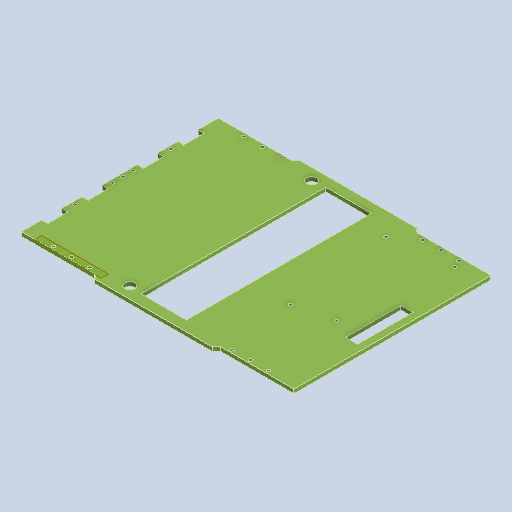
# Autodesk Inventor part: верхняя пластина
Saved by Autodesk Inventor 2024.2 (Build 282272000, 272)
## iProperties
Created: 2025-11-23
Part Number: верхняя пластина
Material: Типовые
Document SubType Name: Modeling
Designer: katya_notebook
Density: 1 g/cm^3
Appearance: Оливково-зеленый
Mass: 177.745 g
Surface Area: 959.322 cm^2
Volume: 177.745 cm^3
Author: katya_notebook
Autodesk Inventor part; units mm, degrees
ref_plane "YZ Plane" through (0, 0, 0) normal (1, 0, 0) x (0, 1, 0)
ref_plane "XZ Plane" through (0, 0, 0) normal (0, 1, 0) x (-1, 0, 0)
ref_plane "XY Plane" through (0, 0, 0) normal (0, 0, 1) x (1, 0, 0)
ref_plane "РабПлоскость1" through (-487.5503, -280.3956, -187.6025) normal (0, -1, 0) x (1, 0, 0)
sketch "Эскиз1" plane through (-487.5503, -280.3956, -187.6025) normal (0, -1, 0) x (1, 0, 0)
  line L0 (-76.4763, 6.5) -> (193.5237, 6.5)
  line L1 (193.5237, 6.5) -> (193.5237, -188.5)
  line L2 (193.5237, -188.5) -> (-76.4763, -188.5)
  line L3 (-76.4763, -188.5) -> (-76.4763, 6.5)
  line L4 (-76.4763, -188.5) -> (-76.4763, -168.5) projected
  circle A0 centre (-12, 3.25) radius 1.75
  circle A1 centre (-48, 3.25) radius 1.75
  circle A2 centre (-30, 3.25) radius 1.75
  line L5 (-76.4763, -91) -> (193.5237, -91)
  circle A3 centre (-12, -185.25) radius 1.75
  circle A4 centre (-48, -185.25) radius 1.75
  circle A5 centre (-30, -185.25) radius 1.75
  point P0 (487.5503, 187.6025)
  point P1 (-60, 3.25)
  dimension "d0" = 195
  dimension "d1" = 270
  dimension "d2" = 0
  dimension "d5" = 3.5
  dimension "d6" = 3.5
  dimension "d8" = 12
  dimension "d9" = 3.25
  dimension "d10" = 3.25
  dimension "d11" = 3.5
  dimension "d12" = 3.25
  dimension "d13" = 18
  dimension "d14" = 97.5
  constraints: 10 end point, 6 centre point, 3 symmetric about line, 2 parallel, 2 perpendicular, 1 horizontal, 1 midpoint, 1 point on line, 3 other
  measures "d0" distance of L0.end L1.end
  measures "d1" distance of L1.end L2.end
  measures "d2" distance between parallel lines of L4 L3
  measures "d5" diameter of A1
  measures "d6" diameter of A0
  measures "d8" distance of A1.centre point (-60, 3.25)
  measures "d9" distance from line of L0 A0.centre
  measures "d10" distance from line of L0 A1.centre
  measures "d11" diameter of A2
  measures "d12" distance from line of L0 A2.centre
  measures "d13" distance of A1.centre A2.centre
  measures "d14" distance between parallel lines of L5 L0
extrude "Выдавливание1" add sketch "Эскиз1" along normal blind 4 contours L0 L1 L5 L3 | L5 L1 L2 L3 | A0 | A1 | A2 | A3 | A4 | A5
sketch "Эскиз2" plane through (-487.5503, -284.3956, -187.6025) normal (0, -1, 0) x (1, 0, 0)
  circle A0 centre (-48, -185.25) radius 1.75 projected
  circle A1 centre (-30, -185.25) radius 1.75 projected
  circle A2 centre (-12, -185.25) radius 1.75 projected
  line L0 (0, -182) -> (-60, -182) projected
  line L1 (-60, -182) -> (-60, -188.5) projected
  line L2 (0, -188.5) -> (-60, -188.5) projected
  line L3 (0, -182) -> (0, -188.5) projected
  circle A3 centre (-48, 3.25) radius 1.75 projected
  circle A4 centre (-30, 3.25) radius 1.75 projected
  circle A5 centre (-12, 3.25) radius 1.75 projected
  line L4 (0, 0) -> (-60, 0) projected
  line L5 (0, 0) -> (0, 6.5) projected
  line L6 (0, 6.5) -> (-60, 6.5) projected
  line L7 (-60, 0) -> (-60, 6.5) projected
  circle A6 centre (165.0475, 3.25) radius 1.75 projected
  circle A7 centre (129.0475, 3.25) radius 1.75 projected
  circle A8 centre (147.0475, 3.25) radius 1.75 projected
  line L8 (116.803, 6.5) -> (116.803, 0) projected
  line L9 (116.803, 0) -> (176.803, 0) projected
  line L10 (176.803, 0) -> (176.803, 6.5) projected
  line L11 (176.803, 6.5) -> (116.803, 6.5) projected
  circle A9 centre (165.0475, -185.25) radius 1.75 projected
  circle A10 centre (129.0475, -185.25) radius 1.75 projected
  circle A11 centre (147.0475, -185.25) radius 1.75 projected
  line L12 (116.803, -188.5) -> (116.803, -182) projected
  line L13 (176.803, -188.5) -> (116.803, -188.5) projected
  line L14 (176.803, -182) -> (176.803, -188.5) projected
  line L15 (116.803, -182) -> (176.803, -182) projected
  line L16 (81.0237, 0.5) -> (81.0237, -182.5) projected
  line L17 (36.0237, 0.5) -> (81.0237, 0.5) projected
  line L18 (36.0237, -182.5) -> (36.0237, 0.5) projected
  line L19 (36.0237, -182.5) -> (81.0237, -182.5) projected
  point P0 (487.5503, 187.6025)
extrude "Выдавливание2" cut sketch "Эскиз2" against normal blind 10 contours A0 | A1 | A2 | A3 | A4 | A5 | A6 | A7 | A8 | A9 | A10 | A11
sketch "Эскиз3" plane through (-487.5503, -284.3956, -187.6025) normal (0, -1, 0) x (1, 0, 0)
  circle A0 centre (23.5237, -1) radius 5 projected
  circle A1 centre (23.5237, -181) radius 5 projected
  line L0 (36.0237, -182.5) -> (36.0237, 0.5) projected
  line L1 (81.0237, 0.5) -> (81.0237, -182.5) projected
  line L2 (36.0237, 0.5) -> (81.0237, 0.5) projected
  line L3 (81.0237, -182.5) -> (36.0237, -182.5) projected
  point P0 (487.5503, 187.6025)
extrude "Выдавливание3" cut sketch "Эскиз3" against normal blind 10
sketch "Эскиз4" plane through (-487.5503, -284.3956, -187.6025) normal (0, -1, 0) x (1, 0, 0)
  arc A0 (116.803, 10.7701) -> (120.803, 6.5) centre (124.2371, 13.7254) ccw projected
  line L0 (116.803, 10.7701) -> (0.2701, 10.7701) projected
  arc A1 (-4, 6.5) -> (0.2701, 10.7701) centre (-7.1034, 13.8735) ccw projected
  arc A2 (0, -192.5) -> (-4, -188.5) centre (-7.2915, -195.7915) ccw projected
  line L1 (0, -192.5) -> (116.803, -192.5) projected
  arc A3 (120.803, -188.5) -> (116.803, -192.5) centre (124.0945, -195.7915) ccw projected
  line L2 (120.803, -188.5) -> (-4, -188.5)
  line L3 (-4, 6.5) -> (120.803, 6.5)
  point P0 (487.5503, 187.6025)
  constraints: 4 end point, 1 horizontal, 1 parallel
extrude "Выдавливание4" add sketch "Эскиз4" against normal blind 4
sketch "Эскиз5" plane through (-487.5503, -284.3956, -187.6025) normal (0, -1, 0) x (1, 0, 0)
  line L0 (174.5237, -118.4235) -> (174.5237, -63.4235) projected
  line L1 (186.5237, -118.4235) -> (174.5237, -118.4235) projected
  line L2 (186.5237, -63.4235) -> (186.5237, -118.4235) projected
  line L3 (174.5237, -63.4235) -> (186.5237, -63.4235) projected
  point P0 (487.5503, 187.6025)
extrude "Выдавливание5" cut sketch "Эскиз5" against normal blind 10
sketch "Эскиз6" plane through (-487.5503, -284.3956, -187.6025) normal (0, -1, 0) x (1, 0, 0)
  circle A0 centre (155.9244, -73.304) radius 1.7 projected
  circle A1 centre (119.3724, -64.137) radius 1.7 projected
  circle A2 centre (108.4264, -169.57) radius 1.7 projected
  circle A3 centre (168.1164, -177.698) radius 1.7 projected
  point P0 (487.5503, 187.6025)
extrude "Выдавливание6" cut sketch "Эскиз6" against normal blind 10
ref_plane "РабПлоскость2" through (-558.0266, -285.3956, -376.1025) normal (1, 0, 0) x (0, 1, 0)
sketch "Эскиз7" plane through (-564.0266, -280.3956, -376.1025) normal (-1, 0, 0) x (0, 0, 1)
  line L0 (175, -5) -> (175, 0) projected
  line L1 (155, 0) -> (155, -5) projected
  line L2 (155, -5) -> (175, -5) projected
  line L3 (195, 0) -> (0, 0) projected
  line L4 (115, -5) -> (135, -5) projected
  line L5 (135, -5) -> (135, 0) projected
  line L6 (115, 0) -> (115, -5) projected
  line L7 (80, -5) -> (80, 0) projected
  line L8 (60, -5) -> (80, -5) projected
  line L9 (60, 0) -> (60, -5) projected
  line L10 (40, -5) -> (40, 0) projected
  line L11 (20, -5) -> (40, -5) projected
  line L12 (20, 0) -> (20, -5) projected
  line L13 (95.75, 39.705) -> (95.75, 46.205) projected
  line L14 (88.875, 55.705) -> (88.875, 49.205) projected
  line L15 (88.875, 49.205) -> (90.375, 49.205) projected
  line L16 (90.375, 49.205) -> (90.375, 46.205) projected
  line L17 (90.375, 46.205) -> (88.875, 46.205) projected
  line L18 (88.875, 39.705) -> (85.375, 39.705) projected
  line L19 (85.375, 39.705) -> (85.375, 46.205) projected
  line L20 (85.375, 46.205) -> (83.875, 46.205) projected
  line L21 (83.875, 46.205) -> (83.875, 49.205) projected
  line L22 (83.875, 49.205) -> (85.375, 49.205) projected
  line L23 (85.375, 49.205) -> (85.375, 55.705) projected
  line L24 (80, 59.705) -> (80, 60.705) projected
  line L25 (80, 60.705) -> (60, 60.705) projected
  line L26 (60, 60.705) -> (60, 59.705) projected
  line L27 (51.75, 55.705) -> (51.75, 49.205) projected
  line L28 (51.75, 49.205) -> (53.25, 49.205) projected
  line L29 (53.25, 49.205) -> (53.25, 46.205) projected
  line L30 (53.25, 46.205) -> (51.75, 46.205) projected
  line L31 (51.75, 39.705) -> (48.25, 39.705) projected
  line L32 (48.25, 39.705) -> (48.25, 46.205) projected
  line L33 (48.25, 46.205) -> (46.75, 46.205) projected
  line L34 (46.75, 46.205) -> (46.75, 49.205) projected
  line L35 (46.75, 49.205) -> (48.25, 49.205) projected
  line L36 (48.25, 49.205) -> (48.25, 55.705) projected
  line L37 (40, 59.705) -> (40, 60.705) projected
  line L38 (40, 60.705) -> (20, 60.705) projected
  line L39 (20, 60.705) -> (20, 59.705) projected
  line L40 (0, 55.705) -> (0, 0) projected
  line L41 (20, 0) -> (0, 0) projected
  line L42 (20, 0) -> (20, -5) projected
  line L43 (20, -5) -> (40, -5) projected
  line L44 (40, -5) -> (40, 0) projected
  line L45 (48.25, 0) -> (40, 0) projected
  line L46 (48.25, 0) -> (48.25, 6.5) projected
  line L47 (48.25, 6.5) -> (46.75, 6.5) projected
  line L48 (46.75, 6.5) -> (46.75, 9.5) projected
  line L49 (46.75, 9.5) -> (48.25, 9.5) projected
  line L50 (48.25, 9.5) -> (48.25, 16) projected
  line L51 (48.25, 16) -> (51.75, 16) projected
  line L52 (51.75, 16) -> (51.75, 9.5) projected
  line L53 (51.75, 9.5) -> (53.25, 9.5) projected
  line L54 (53.25, 9.5) -> (53.25, 6.5) projected
  line L55 (53.25, 6.5) -> (51.75, 6.5) projected
  line L56 (51.75, 6.5) -> (51.75, 0) projected
  line L57 (60, 0) -> (51.75, 0) projected
  line L58 (60, 0) -> (60, -5) projected
  line L59 (60, -5) -> (80, -5) projected
  line L60 (80, -5) -> (80, 0) projected
  line L61 (85.375, 0) -> (80, 0) projected
  line L62 (85.375, 0) -> (85.375, 6.5) projected
  line L63 (85.375, 6.5) -> (83.875, 6.5) projected
  line L64 (83.875, 6.5) -> (83.875, 9.5) projected
  line L65 (83.875, 9.5) -> (85.375, 9.5) projected
  line L66 (85.375, 9.5) -> (85.375, 16) projected
  line L67 (85.375, 16) -> (88.875, 16) projected
  line L68 (88.875, 16) -> (88.875, 9.5) projected
  line L69 (88.875, 9.5) -> (90.375, 9.5) projected
  line L70 (90.375, 9.5) -> (90.375, 6.5) projected
  line L71 (90.375, 6.5) -> (88.875, 6.5) projected
  line L72 (88.875, 6.5) -> (88.875, 0) projected
  line L73 (95.75, 0) -> (88.875, 0) projected
  line L74 (95.75, 0) -> (95.75, 6.5) projected
  line L75 (95.75, 6.5) -> (94.25, 6.5) projected
  line L76 (94.25, 6.5) -> (94.25, 9.5) projected
  line L77 (94.25, 9.5) -> (95.75, 9.5) projected
  line L78 (95.75, 9.5) -> (95.75, 16) projected
  line L79 (95.75, 16) -> (99.25, 16) projected
  line L80 (99.25, 16) -> (99.25, 9.5) projected
  line L81 (99.25, 9.5) -> (100.75, 9.5) projected
  line L82 (100.75, 9.5) -> (100.75, 6.5) projected
  line L83 (100.75, 6.5) -> (99.25, 6.5) projected
  line L84 (99.25, 6.5) -> (99.25, 0) projected
  line L85 (106.125, 0) -> (99.25, 0) projected
  line L86 (106.125, 0) -> (106.125, 6.5) projected
  line L87 (106.125, 6.5) -> (104.625, 6.5) projected
  line L88 (104.625, 6.5) -> (104.625, 9.5) projected
  line L89 (104.625, 9.5) -> (106.125, 9.5) projected
  line L90 (106.125, 9.5) -> (106.125, 16) projected
  line L91 (106.125, 16) -> (109.625, 16) projected
  line L92 (109.625, 16) -> (109.625, 9.5) projected
  line L93 (109.625, 9.5) -> (111.125, 9.5) projected
  line L94 (111.125, 9.5) -> (111.125, 6.5) projected
  line L95 (111.125, 6.5) -> (109.625, 6.5) projected
  line L96 (109.625, 6.5) -> (109.625, 0) projected
  line L97 (115, 0) -> (109.625, 0) projected
  line L98 (115, 0) -> (115, -5) projected
  line L99 (115, -5) -> (135, -5) projected
  line L100 (135, -5) -> (135, 0) projected
  line L101 (143.25, 0) -> (135, 0) projected
  line L102 (143.25, 0) -> (143.25, 6.5) projected
  line L103 (143.25, 6.5) -> (141.75, 6.5) projected
  line L104 (141.75, 6.5) -> (141.75, 9.5) projected
  line L105 (141.75, 9.5) -> (143.25, 9.5) projected
  line L106 (143.25, 9.5) -> (143.25, 16) projected
  line L107 (143.25, 16) -> (146.75, 16) projected
  line L108 (146.75, 16) -> (146.75, 9.5) projected
  line L109 (146.75, 9.5) -> (148.25, 9.5) projected
  line L110 (148.25, 9.5) -> (148.25, 6.5) projected
  line L111 (148.25, 6.5) -> (146.75, 6.5) projected
  line L112 (146.75, 6.5) -> (146.75, 0) projected
  line L113 (155, 0) -> (146.75, 0) projected
  line L114 (155, 0) -> (155, -5) projected
  line L115 (155, -5) -> (175, -5) projected
  line L116 (175, -5) -> (175, 0) projected
  line L117 (195, 0) -> (175, 0) projected
  line L118 (195, 55.705) -> (195, 0) projected
  line L119 (175, 59.705) -> (175, 60.705) projected
  line L120 (175, 60.705) -> (155, 60.705) projected
  line L121 (155, 60.705) -> (155, 59.705) projected
  line L122 (146.75, 55.705) -> (146.75, 49.205) projected
  line L123 (146.75, 49.205) -> (148.25, 49.205) projected
  line L124 (148.25, 49.205) -> (148.25, 46.205) projected
  line L125 (148.25, 46.205) -> (146.75, 46.205) projected
  line L126 (146.75, 46.205) -> (146.75, 39.705) projected
  line L127 (146.75, 39.705) -> (143.25, 39.705) projected
  line L128 (143.25, 39.705) -> (143.25, 46.205) projected
  line L129 (143.25, 46.205) -> (141.75, 46.205) projected
  line L130 (141.75, 46.205) -> (141.75, 49.205) projected
  line L131 (141.75, 49.205) -> (143.25, 49.205) projected
  line L132 (143.25, 49.205) -> (143.25, 55.705) projected
  line L133 (135, 59.705) -> (135, 60.705) projected
  line L134 (135, 60.705) -> (115, 60.705) projected
  line L135 (115, 60.705) -> (115, 59.705) projected
  line L136 (109.625, 55.705) -> (109.625, 49.205) projected
  line L137 (109.625, 49.205) -> (111.125, 49.205) projected
  line L138 (111.125, 49.205) -> (111.125, 46.205) projected
  line L139 (111.125, 46.205) -> (109.625, 46.205) projected
  line L140 (109.625, 46.205) -> (109.625, 39.705) projected
  line L141 (109.625, 39.705) -> (106.125, 39.705) projected
  line L142 (106.125, 39.705) -> (106.125, 46.205) projected
  line L143 (106.125, 46.205) -> (104.625, 46.205) projected
  line L144 (104.625, 46.205) -> (104.625, 49.205) projected
  line L145 (104.625, 49.205) -> (106.125, 49.205) projected
  line L146 (106.125, 49.205) -> (106.125, 55.705) projected
  line L147 (99.25, 55.705) -> (99.25, 49.205) projected
  line L148 (99.25, 49.205) -> (100.75, 49.205) projected
  line L149 (100.75, 49.205) -> (100.75, 46.205) projected
  line L150 (100.75, 46.205) -> (99.25, 46.205) projected
  line L151 (99.25, 39.705) -> (95.75, 39.705) projected
  line L152 (95.75, 46.205) -> (94.25, 46.205) projected
  line L153 (94.25, 46.205) -> (94.25, 49.205) projected
  line L154 (94.25, 49.205) -> (95.75, 49.205) projected
  line L155 (0, 55.705) -> (20, 55.705) projected
  line L156 (51.75, 46.205) -> (51.75, 39.705) projected
  line L157 (88.875, 46.205) -> (88.875, 39.705) projected
  line L158 (95.75, 49.205) -> (95.75, 55.705) projected
  line L159 (99.25, 46.205) -> (99.25, 39.705) projected
  line L160 (115, 55.705) -> (109.625, 55.705) projected
  line L161 (106.125, 55.705) -> (99.25, 55.705) projected
  line L162 (95.75, 55.705) -> (88.875, 55.705) projected
  line L163 (85.375, 55.705) -> (80, 55.705) projected
  line L164 (80, 55.705) -> (80, 59.705) projected
  line L165 (60, 59.705) -> (60, 55.705) projected
  line L166 (60, 55.705) -> (51.75, 55.705) projected
  line L167 (48.25, 55.705) -> (40, 55.705) projected
  line L168 (40, 55.705) -> (40, 59.705) projected
  line L169 (20, 59.705) -> (20, 55.705) projected
  line L170 (20, 55.705) -> (0, 55.705) projected
  line L171 (195, 55.705) -> (175, 55.705) projected
  line L172 (175, 55.705) -> (175, 59.705) projected
  line L173 (155, 59.705) -> (155, 55.705) projected
  line L174 (155, 55.705) -> (146.75, 55.705) projected
  line L175 (143.25, 55.705) -> (135, 55.705) projected
  line L176 (135, 55.705) -> (135, 59.705) projected
  line L177 (115, 59.705) -> (115, 55.705) projected
  point P0 (376.1025, 280.3956)
  point P1 (155, 55.705)
  point P2 (175, 55.705)
  point P3 (115, 55.705)
  point P4 (135, 55.705)
  point P5 (60, 55.705)
  point P6 (80, 55.705)
  point P7 (40, 55.705)
  point P8 (20, 0)
  point P9 (40, 0)
  point P10 (60, 0)
  point P11 (80, 0)
  point P12 (135, 0)
  point P13 (46.75, 47.1901)
  dimension "d0" = 195
  dimension "d1" = 270
  dimension "d2" = 0
  dimension "d5" = 3.5
  dimension "d6" = 3.5
  dimension "d8" = 12
  dimension "d9" = 3.25
  dimension "d10" = 3.25
  dimension "d11" = 3.5
  dimension "d12" = 3.25
  dimension "d13" = 18
  dimension "d14" = 97.5
extrude "Выдавливание7" cut sketch "Эскиз7" against normal up to surface (6 mm away) contours L2 L1 L3 L0 | L5 L4 L6 L3 | L7 L8 L9 L3 | L10 L11 L12 L3
sketch "Эскиз8" plane through (-487.5503, -284.3956, -187.6025) normal (0, -1, 0) x (1, 0, 0)
  line L0 (-70.4763, -45.25) -> (-76.4763, -45.25)
  line L1 (-76.4763, -40.25) -> (-70.4763, -40.25)
  line L2 (-76.4763, -45.25) -> (-76.4763, -41.75)
  line L3 (-76.4763, -45.25) -> (-70.4763, -45.25)
  line L4 (-70.4763, -41.75) -> (-70.4763, -45.25)
  line L5 (-76.4763, -41.75) -> (-70.4763, -41.75)
  line L6 (-76.4763, -82.375) -> (-76.4763, -78.875)
  line L7 (-76.4763, -82.375) -> (-70.4763, -82.375)
  line L8 (-70.4763, -78.875) -> (-70.4763, -82.375)
  line L9 (-76.4763, -78.875) -> (-70.4763, -78.875)
  line L10 (-76.4763, -92.75) -> (-76.4763, -89.25)
  line L11 (-76.4763, -92.75) -> (-70.4763, -92.75)
  line L12 (-70.4763, -89.25) -> (-70.4763, -92.75)
  line L13 (-76.4763, -89.25) -> (-70.4763, -89.25)
  line L14 (-76.4763, -103.125) -> (-76.4763, -99.625)
  line L15 (-76.4763, -103.125) -> (-70.4763, -103.125)
  line L16 (-70.4763, -99.625) -> (-70.4763, -103.125)
  line L17 (-76.4763, -99.625) -> (-70.4763, -99.625)
  line L18 (-76.4763, -140.25) -> (-76.4763, -136.75)
  line L19 (-76.4763, -140.25) -> (-70.4763, -140.25)
  line L20 (-70.4763, -136.75) -> (-70.4763, -140.25)
  line L21 (-76.4763, -136.75) -> (-70.4763, -136.75)
  circle A0 centre (-73.4763, -43.5) radius 1.75
  circle A1 centre (-73.4763, -80.625) radius 1.75
  circle A2 centre (-73.4763, -91) radius 1.75
  circle A3 centre (-73.4763, -101.375) radius 1.75
  circle A4 centre (-73.4763, -138.5) radius 1.75
  point P0 (487.5503, 187.6025)
extrude "Выдавливание8" cut sketch "Эскиз8" against normal blind 10 contours A0 | A1 | A2 | A3 | A4
